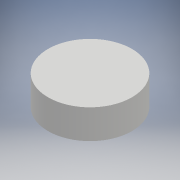
# Autodesk Inventor part: Support pasApas
Saved by Autodesk Inventor 2018 (Build 220112000, 112)
## iProperties
Created: 2018-03-31
Part Number: Support pasApas
Material: Générique
Document SubType Name: Modeling
Designer: Guadalix
Density: 1 g/cm^3
Appearance: Par défaut
Author: Guadalix
Autodesk Inventor part; units mm, degrees
ref_plane "YZ Plane" through (0, 0, 0) normal (1, 0, 0) x (0, 1, 0)
ref_plane "XZ Plane" through (0, 0, 0) normal (0, 1, 0) x (-1, 0, 0)
ref_plane "XY Plane" through (0, 0, 0) normal (0, 0, 1) x (1, 0, 0)
sketch "Esquisse1" plane through (0, 0, 0) normal (0, 0, 1) x (1, 0, 0)
  circle A0 centre (0, 0) radius 20.5
  circle A1 centre (0, 0) radius 21.5
  line L0 (0.7498, -6.187) -> (-0.7498, -6.187)
  line L1 (-0.7498, -6.187) -> (-0.7498, 6.187)
  line L2 (-0.7498, 6.187) -> (0.7498, 6.187)
  line L3 (0.7498, 6.187) -> (0.7498, -6.187)
  line L4 (0.7498, -6.187) -> (-0.7498, 6.187) construction
  line L5 (-0.7498, -6.187) -> (0.7498, 6.187) construction
  point P0 (20.5, 0)
  point P1 (21.5, 0)
  dimension "d0" = 41
  dimension "d1" = 43
  dimension "d16" = 1
  constraints: 12 end point, 2 coincident, 2 horizontal alignment, 2 midpoint, 2 parallel, 1 horizontal, 1 perpendicular, 4 other
  measures "d16" distance of point (21.5, 0) point (20.5, 0)
extrude "Extrusion1" add sketch "Esquisse1" along normal blind 15 contours A1
sketch "Esquisse2" plane through (0, 0, 15) normal (0, 0, 1) x (1, 0, 0)
  circle A0 centre (0, 0) radius 20.5
  constraints: 1 centre point, 1 coincident
extrude "Extrusion2" add sketch "Esquisse2" against normal blind 5
sketch "Esquisse3" plane through (0, 0, 10) normal (0, 0, -1) x (-1, 0, 0)
  line L0 (1.65, 6) -> (-1.65, 6)
  line L1 (-1.65, 6) -> (-1.65, -6)
  line L2 (-1.65, -6) -> (1.65, -6)
  line L3 (1.65, -6) -> (1.65, 6)
  line L4 (1.65, 6) -> (-1.65, -6) construction
  line L5 (-1.65, 6) -> (1.65, -6) construction
  point P0 (0, 0)
  dimension "d8" = 12
  dimension "d9" = 3.3
  constraints: 12 end point, 2 midpoint, 2 parallel, 1 horizontal, 1 perpendicular
  measures "d8" distance of L2.end L0.start
  measures "d9" distance of L1.end L2.end
extrude "Extrusion3" cut sketch "Esquisse3" against normal blind 4
